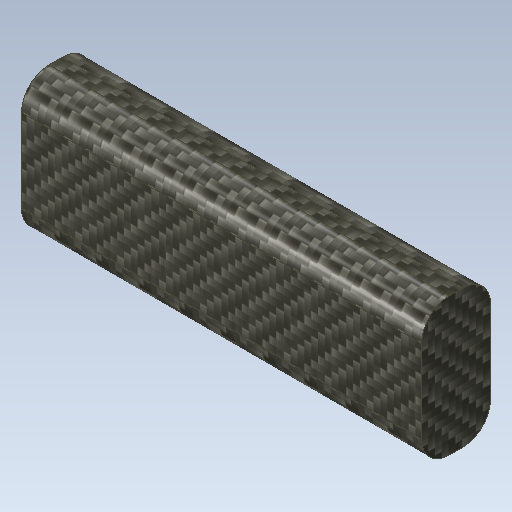
# Autodesk Inventor part: バッテリー
Saved by Autodesk Inventor 2020 (Build 240168000, 168)
## iProperties
Part Number: バッテリー
Material: 一般
Document SubType Name: Modeling
Designer: tanjihayato
Mass: 170 g
Surface Area: 235 cm^2
Volume: 175 cm^3
Density: 0.971429 g/cm^3
Appearance: カーボンファイバー 1
Author: tanjihayato
Autodesk Inventor part; units mm, degrees
ref_plane "YZ Plane" through (0, 0, 0) normal (1, 0, 0) x (0, 1, 0)
ref_plane "XZ Plane" through (0, 0, 0) normal (0, 1, 0) x (-1, 0, 0)
ref_plane "XY Plane" through (0, 0, 0) normal (0, 0, 1) x (1, 0, 0)
sketch "スケッチ1" plane through (0, 0, 0) normal (0, 0, 1) x (1, 0, 0)
  line L0 (-18.0483, 45.0034) -> (126.9517, 45.0034)
  line L1 (126.9517, 45.0034) -> (126.9517, -4.9966)
  line L2 (126.9517, -4.9966) -> (-18.0483, -4.9966)
  line L3 (-18.0483, -4.9966) -> (-18.0483, 45.0034)
  point P0 (0, 0)
  dimension "d0" = 145
  dimension "d1" = 50
  constraints: 8 end point, 2 parallel, 1 horizontal, 1 perpendicular
  measures "d0" distance of L1.end L2.end
  measures "d1" distance of L0.end L1.end
extrude "押し出し1" add sketch "スケッチ1" along normal blind 25
fillet "フィレット1" radius 10 4 edges at (54.4517, 45.0034, 25) (54.4517, 45.0034, 0) (54.4517, -4.9966, 25) (54.4517, -4.9966, 0)
